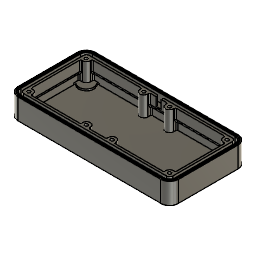
Case Bottom (Autodesk Fusion 360 design; units mm, degrees)
Autodesk Fusion 360 part; units mm, degrees
sketch "Sketch1" plane through (0, 0, 0) normal (0, 0, 1) x (1, 0, 0)
  line L0 (2, 0) -> (146, 0)
  line L1 (148, 2) -> (148, 62)
  line L2 (146, 64) -> (2, 64)
  line L3 (0, 62) -> (0, 2)
  arc A0 (2, 64) -> (0, 62) centre (2, 62) ccw
  arc A1 (0, 2) -> (2, 0) centre (2, 2) ccw
  arc A2 (146, 0) -> (148, 2) centre (146, 2) ccw
  arc A3 (148, 62) -> (146, 64) centre (146, 62) ccw
  line L4 (-0.4, 62) -> (-0.4, 2)
  arc A4 (-0.4, 2) -> (2, -0.4) centre (2, 2) ccw
  line L5 (2, -0.4) -> (146, -0.4)
  arc A5 (146, -0.4) -> (148.4, 2) centre (146, 2) ccw
  line L6 (148.4, 2) -> (148.4, 62)
  arc A6 (148.4, 62) -> (146, 64.4) centre (146, 62) ccw
  line L7 (146, 64.4) -> (2, 64.4)
  arc A7 (2, 64.4) -> (-0.4, 62) centre (2, 62) ccw
  circle A8 centre (3, 61) radius 4
  circle A9 centre (61, 61) radius 4
  circle A10 centre (87, 61) radius 4
  circle A11 centre (3, 3) radius 4
  circle A12 centre (61, 3) radius 4
  circle A13 centre (87, 3) radius 4
  circle A14 centre (145, 3) radius 4
  circle A15 centre (145, 61) radius 4
  line L8 (7, 61) -> (7, 64.4)
  line L9 (3, 57) -> (-0.4, 57)
  line L10 (57, 61) -> (57, 62)
  line L11 (57, 62) -> (57, 64.4)
  line L12 (65, 61) -> (65, 62.4151)
  line L13 (65, 62.4151) -> (65, 64.4)
  line L14 (83, 61) -> (83, 64.4)
  line L15 (91, 61) -> (91, 64.4)
  line L16 (141, 61) -> (141, 64.4)
  line L17 (145, 57) -> (148.4, 57)
  line L18 (145, 7) -> (148.4, 7)
  line L19 (141, 3) -> (141, -0.4)
  line L20 (91, 3) -> (91, -0.4)
  line L21 (83, 3) -> (83, -0.4)
  line L22 (65, 3) -> (65, -0.4)
  line L23 (57, 3) -> (57, -0.4)
  line L24 (7, 3) -> (7, -0.4)
  line L25 (3, 7) -> (-0.4, 7)
  line L26 (-7, 62) -> (-7, 2)
  arc A16 (-7, 2) -> (2, -7) centre (2, 2) ccw
  line L27 (2, -7) -> (146, -7)
  arc A17 (146, -7) -> (155, 2) centre (146, 2) ccw
  line L28 (155, 2) -> (155, 62)
  arc A18 (155, 62) -> (146, 71) centre (146, 62) ccw
  line L29 (146, 71) -> (2, 71)
  arc A19 (2, 71) -> (-7, 62) centre (2, 62) ccw
  point P0 (148, 0)
  point P1 (0, 64)
  point P2 (3, 61)
  point P3 (3, 3)
  point P4 (61, 3)
  point P5 (87, 3)
  point P6 (145, 3)
  point P7 (61, 61)
  point P8 (87, 61)
  point P9 (145, 61)
  dimension "d1" = 148
  dimension "d2" = 64
  dimension "d3" = 2
  dimension "d4" = 0.4
  dimension "d5" = 3
  dimension "d6" = 3
  dimension "d7" = 3
  dimension "d8" = 58
  dimension "d9" = 3
  dimension "d10" = 58
  dimension "d11" = 3
  dimension "d12" = 3
  dimension "d13" = 3
  dimension "d14" = 3
  dimension "d15" = 3
  dimension "d16" = 3
  dimension "d17" = 58
  dimension "d18" = 3
  dimension "d19" = 3
  dimension "d20" = 58
  dimension "d21" = 8
  dimension "d22" = 8
  dimension "d23" = 8
  dimension "d24" = 8
  dimension "d25" = 8
  dimension "d26" = 8
  dimension "d27" = 8
  dimension "d28" = 8
  dimension "d96" = 7
  constraint horizontal L0
  constraint vertical L1
  constraint horizontal L2
  constraint vertical L3
  constraint coincident P1 L3
  constraint coincident P1 L2
  constraint tangent L3 A0
  constraint tangent L2 A0
  constraint coincident origin L3
  constraint coincident origin L0
  constraint tangent L3 A1
  constraint tangent L0 A1
  constraint equal A0 A1
  constraint coincident P0 L1
  constraint coincident P0 L0
  constraint tangent L1 A2
  constraint tangent L0 A2
  constraint equal A0 A2
  constraint tangent L1 A3
  constraint tangent L2 A3
  constraint equal A0 A3
  constraint coincident P2 A8.centre
  constraint coincident P7 A9.centre
  constraint coincident P8 A10.centre
  constraint coincident P3 A11.centre
  constraint coincident P4 A12.centre
  constraint coincident P5 A13.centre
  constraint coincident P6 A14.centre
  constraint coincident P9 A15.centre
  constraint coincident A8 L8.start
  constraint coincident L7 L8.end
  constraint perpendicular L7 L8
  constraint tangent A8 L8
  constraint coincident A8 L9.start
  constraint coincident L4 L9.end
  constraint perpendicular L4 L9
  constraint tangent A8 L9
  constraint coincident A9 L10.start
  constraint tangent A9 L10
  constraint perpendicular L9 L10
  constraint coincident L7 L11.end
  constraint perpendicular L7 L11
  constraint coincident A9 L12.start
  constraint tangent A9 L12
  constraint perpendicular L7 L12
  constraint coincident L7 L13.end
  constraint perpendicular L7 L13
  constraint coincident A10 L14.start
  constraint coincident L7 L14.end
  constraint perpendicular L7 L14
  constraint coincident A10 L15.start
  constraint coincident L7 L15.end
  constraint perpendicular L7 L15
  constraint tangent A10 L14
  constraint tangent A10 L15
  constraint coincident A15 L16.start
  constraint coincident L7 L16.end
  constraint perpendicular L7 L16
  constraint coincident A15 L17.start
  constraint coincident L6 L17.end
  constraint perpendicular L6 L17
  constraint tangent A15 L16
  constraint tangent A15 L17
  constraint coincident A14 L18.start
  constraint coincident L6 L18.end
  constraint tangent A14 L18
  constraint coincident A14 L19.start
  constraint coincident L5 L19.end
  constraint perpendicular L5 L19
  constraint coincident A13 L20.start
  constraint coincident L5 L20.end
  constraint perpendicular L5 L20
  constraint coincident A13 L21.start
  constraint coincident L5 L21.end
  constraint perpendicular L5 L21
  constraint tangent A13 L20
  constraint tangent A13 L21
  constraint tangent A14 L19
  constraint perpendicular L6 L18
  constraint coincident A12 L22.start
  constraint coincident L5 L22.end
  constraint perpendicular L5 L22
  constraint coincident A12 L23.start
  constraint coincident L5 L23.end
  constraint perpendicular L5 L23
  constraint tangent A12 L22
  constraint tangent A12 L23
  constraint coincident A11 L24.start
  constraint coincident L5 L24.end
  constraint perpendicular L5 L24
  constraint coincident A11 L25.start
  constraint coincident L4 L25.end
  constraint perpendicular L4 L25
  constraint tangent A11 L25
  constraint tangent A11 L24
  measures "d1" distance of origin P0
  measures "d2" distance of origin P1
  measures "d3" radius of A0
  measures "d5" distance of L3 P2
  measures "d6" distance of L2 P2
  measures "d7" distance of L2 P7
  measures "d8" distance of P2 P7
  measures "d9" distance of L2 P8
  measures "d10" horizontal distance of P8 P9
  measures "d11" distance of L2 P9
  measures "d12" distance of L1 P9
  measures "d13" distance of L0 P6
  measures "d14" distance of L1 P6
  measures "d15" distance of L0 P5
  measures "d16" distance of L0 P4
  measures "d17" horizontal distance of P3 P4
  measures "d18" distance of L3 P3
  measures "d19" distance of L0 P3
  measures "d20" distance of P5 P6
  measures "d21" diameter of A8
  measures "d22" diameter of A9
  measures "d23" diameter of A10
  measures "d24" diameter of A11
  measures "d25" diameter of A12
  measures "d26" diameter of A13
  measures "d27" diameter of A14
  measures "d28" diameter of A15
extrude "Extrude1" add sketch "Sketch1" along normal blind 20 contours L0 L3 A1 A11 | L0 L3 A1 L4 A4 L5 A11 | L0 A11 L24 | L0 L5 A11 L24 | L4 A4 L5 A11 | L3 L4 A11 L25 | L3 A11 L25 | L0 A12 L23 | L0 L5 A12 L23 | L0 A12 | L0 L5 A12 | L3 L4 A8 L9 | L3 A8 L9 | L0 A12 L22 | L0 L5 A12 L22 | L5 A12 | L2 L3 A0 L4 L7 A7 A8 | L2 L3 A0 A8 | L4 L7 A7 A8 | L2 A8 L8 | L0 A13 L21 | L0 L5 A13 L21 | L2 L7 A8 L8 | L0 A13 | L0 L5 A13 | L2 L7 A9 L11 | L2 A9 L10 L11 | L0 A13 L20 | L0 L5 A13 L20 | L5 A13 | L2 L7 A9 | L2 A9 | L7 A9 | L2 L7 A9 L13 | L2 A9 L12 L13 | L0 A14 L19 | L0 L5 A14 L19 | L0 L1 A2 A14 | L0 L1 A2 L5 A5 L6 A14 | L2 L7 A10 L14 | L2 A10 L14 | L5 A5 L6 A14 | L1 A14 L18 | L2 L7 A10 | L2 A10 | L1 L6 A14 L18 | L7 A10 | L2 L7 A10 L15 | L2 A10 L15 | L1 A15 L17 | L1 L6 A15 L17 | L1 L2 A3 A15 | L1 L2 A3 L6 A6 L7 A15 | L2 L7 A15 L16 | L2 A15 L16 | L6 A6 L7 A15 | L26 A16 L27 A17 L28 A18 L29 A19
sketch "PCB Reference" plane through (0, 0, 20) normal (0, 0, 1) x (-1, 0, 0)
  line L0 (-7, 0.4) -> (-7, -3)
  arc A0 (-7, -3) -> (-3, -7) centre (-3, -3) ccw
  line L1 (-3, -7) -> (0.4, -7)
  line L2 (0.4, -7) -> (0.4, -57)
  line L3 (0.4, -57) -> (-3, -57)
  arc A1 (-3, -57) -> (-7, -61) centre (-3, -61) ccw
  line L4 (-7, -61) -> (-7, -64.4)
  line L5 (-7, -64.4) -> (-57, -64.4)
  line L6 (-57, -64.4) -> (-57, -61)
  arc A2 (-57, -61) -> (-65, -61) centre (-61, -61) ccw
  line L7 (-65, -61) -> (-65, -64.4)
  line L8 (-65, -64.4) -> (-83, -64.4)
  line L9 (-83, -64.4) -> (-83, -61)
  arc A3 (-83, -61) -> (-91, -61) centre (-87, -61) ccw
  line L10 (-91, -61) -> (-91, -64.4)
  line L11 (-91, -64.4) -> (-141, -64.4)
  line L12 (-141, 0.4) -> (-91, 0.4)
  line L13 (-91, 0.4) -> (-91, -3)
  arc A4 (-91, -3) -> (-83, -3) centre (-87, -3) ccw
  line L14 (-83, -3) -> (-83, 0.4)
  line L15 (-83, 0.4) -> (-65, 0.4)
  line L16 (-65, 0.4) -> (-65, -3)
  arc A5 (-65, -3) -> (-57, -3) centre (-61, -3) ccw
  line L17 (-57, -3) -> (-57, 0.4)
  line L18 (-57, 0.4) -> (-7, 0.4)
  line L19 (-2, -64) -> (-146, -64)
  line L20 (-148, -62) -> (-148, -2)
  line L21 (-146, 0) -> (-2, 0)
  line L22 (0, -2) -> (0, -62)
  arc A6 (-2, -64) -> (0, -62) centre (-2, -62) ccw
  arc A7 (0, -2) -> (-2, 0) centre (-2, -2) ccw
  arc A8 (-146, 0) -> (-148, -2) centre (-146, -2) ccw
  arc A9 (-148, -62) -> (-146, -64) centre (-146, -62) ccw
  arc A10 (-148.4, -62) -> (-146, -64.4) centre (-146, -62) ccw
  line L23 (-2, -64.4) -> (-146, -64.4)
  arc A11 (-2, -64.4) -> (0.4, -62) centre (-2, -62) ccw
  line L24 (0.4, -2) -> (0.4, -62)
  arc A12 (0.4, -2) -> (-2, 0.4) centre (-2, -2) ccw
  line L25 (-146, 0.4) -> (-2, 0.4)
  arc A13 (-146, 0.4) -> (-148.4, -2) centre (-146, -2) ccw
  line L26 (-148.4, -62) -> (-148.4, -2)
  line L27 (6.4, -70.4) -> (-154.4, -70.4)
  line L28 (-154.4, -70.4) -> (-154.4, 6.4)
  line L29 (-154.4, 6.4) -> (6.4, 6.4)
  line L30 (6.4, 6.4) -> (6.4, -70.4)
  line L31 (-141, -64.4) -> (-141, -61)
  arc A14 (-141, -61) -> (-145, -57) centre (-145, -61) ccw
  line L32 (-145, -57) -> (-148.4, -57)
  line L33 (-148.4, -57) -> (-148.4, -7)
  line L34 (-148.4, -7) -> (-145, -7)
  arc A15 (-145, -7) -> (-141, -3) centre (-145, -3) ccw
  line L35 (-141, -3) -> (-141, 0.4)
  arc A16 (-2, -71) -> (7, -62) centre (-2, -62) ccw
  line L36 (7, -62) -> (7, -2)
  arc A17 (7, -2) -> (-2, 7) centre (-2, -2) ccw
  line L37 (-2, 7) -> (-146, 7)
  arc A18 (-146, 7) -> (-155, -2) centre (-146, -2) ccw
  line L38 (-155, -2) -> (-155, -62)
  arc A19 (-155, -62) -> (-146, -71) centre (-146, -62) ccw
  line L39 (-146, -71) -> (-2, -71)
  point P0 (0, -64)
  point P1 (-148, -64)
  dimension "d36" = 64.8
  dimension "d37" = 148
  dimension "d38" = 64
  dimension "d39" = 0.4
  dimension "d40" = 0.4
  dimension "d41" = 2
  dimension "d42" = -0.4
  constraint horizontal L19
  constraint vertical L20
  constraint horizontal L21
  constraint vertical L22
  constraint coincident P0 L19
  constraint coincident P0 L22
  constraint tangent L19 A6
  constraint tangent L22 A6
  constraint coincident origin L22
  constraint coincident origin L21
  constraint tangent L22 A7
  constraint tangent L21 A7
  constraint equal A6 A7
  constraint tangent L21 A8
  constraint tangent L20 A8
  constraint equal A6 A8
  constraint coincident P1 L20
  constraint coincident P1 L19
  constraint tangent L20 A9
  constraint tangent L19 A9
  constraint equal A6 A9
  constraint horizontal L27
  constraint vertical L28
  constraint horizontal L29
  constraint vertical L30
  measures "d36" distance of L5 L18
  measures "d37" distance of P0 P1
  measures "d38" distance of P0 origin
  measures "d39" distance of L5 L19
  measures "d40" distance of L2 L22
  measures "d41" radius of A6
sketch "Sketch3" plane through (0, 0, 20) normal (0, 0, 1) x (-1, 0, 0)
  line L0 (-7, -64.4) -> (-57, -64.4)
  line L1 (0.4, -7) -> (0.4, -57)
  line L2 (0.4, -57) -> (-3, -57)
  arc A0 (-3, -57) -> (-7, -61) centre (-3, -61) ccw
  line L3 (-7, -61) -> (-7, -64.4)
  circle A1 centre (-3, -61) radius 2
  circle A2 centre (-61, -61) radius 2
  arc A3 (-57, -61) -> (-65, -61) centre (-61, -61) ccw
  circle A4 centre (-87, -61) radius 2
  arc A5 (-83, -61) -> (-91, -61) centre (-87, -61) ccw
  circle A6 centre (-145, -61) radius 2
  arc A7 (-141, -61) -> (-145, -57) centre (-145, -61) ccw
  circle A8 centre (-145, -3) radius 2
  arc A9 (-145, -7) -> (-141, -3) centre (-145, -3) ccw
  circle A10 centre (-87, -3) radius 2
  arc A11 (-91, -3) -> (-83, -3) centre (-87, -3) ccw
  circle A12 centre (-61, -3) radius 2
  arc A13 (-65, -3) -> (-57, -3) centre (-61, -3) ccw
  circle A14 centre (-3, -3) radius 2
  arc A15 (-7, -3) -> (-3, -7) centre (-3, -3) ccw
  line L4 (-7, 0.4) -> (-7, -3)
  arc A16 (-7, -3) -> (-3, -7) centre (-3, -3) ccw
  line L5 (-3, -7) -> (0.4, -7)
  line L6 (-57, -64.4) -> (-57, -61)
  arc A17 (-57, -61) -> (-65, -61) centre (-61, -61) ccw
  line L7 (-65, -61) -> (-65, -64.4)
  line L8 (-65, -64.4) -> (-83, -64.4)
  line L9 (-83, -64.4) -> (-83, -61)
  arc A18 (-83, -61) -> (-91, -61) centre (-87, -61) ccw
  line L10 (-91, -61) -> (-91, -64.4)
  line L11 (-91, -64.4) -> (-141, -64.4)
  line L12 (-141, -64.4) -> (-141, -61)
  arc A19 (-141, -61) -> (-145, -57) centre (-145, -61) ccw
  line L13 (-145, -57) -> (-148.4, -57)
  line L14 (-148.4, -57) -> (-148.4, -7)
  line L15 (-148.4, -7) -> (-145, -7)
  arc A20 (-145, -7) -> (-141, -3) centre (-145, -3) ccw
  line L16 (-141, -3) -> (-141, 0.4)
  line L17 (-141, 0.4) -> (-91, 0.4)
  line L18 (-91, 0.4) -> (-91, -3)
  arc A21 (-91, -3) -> (-83, -3) centre (-87, -3) ccw
  line L19 (-83, -3) -> (-83, 0.4)
  line L20 (-83, 0.4) -> (-65, 0.4)
  line L21 (-65, 0.4) -> (-65, -3)
  arc A22 (-65, -3) -> (-57, -3) centre (-61, -3) ccw
  line L22 (-57, -3) -> (-57, 0.4)
  line L23 (-57, 0.4) -> (-7, 0.4)
  arc A23 (-2, -71) -> (7, -62) centre (-2, -62) ccw
  line L24 (7, -62) -> (7, -2)
  arc A24 (7, -2) -> (-2, 7) centre (-2, -2) ccw
  line L25 (-2, 7) -> (-146, 7)
  arc A25 (-146, 7) -> (-155, -2) centre (-146, -2) ccw
  line L26 (-155, -2) -> (-155, -62)
  arc A26 (-155, -62) -> (-146, -71) centre (-146, -62) ccw
  line L27 (-146, -71) -> (-2, -71)
  dimension "d49" = 4
  dimension "d50" = 4
  dimension "d51" = 4
  dimension "d52" = 4
  dimension "d53" = 4
  dimension "d54" = 4
  dimension "d55" = 4
  dimension "d56" = 4
  constraint concentric A0 A1
  constraint concentric A2 A3
  constraint concentric A4 A5
  constraint concentric A6 A7
  constraint concentric A8 A9
  constraint concentric A10 A11
  constraint concentric A12 A13
  constraint concentric A14 A15
  measures "d49" diameter of A1
  measures "d50" diameter of A2
  measures "d51" diameter of A4
  measures "d52" diameter of A6
  measures "d53" diameter of A8
  measures "d54" diameter of A10
  measures "d55" diameter of A12
  measures "d56" diameter of A14
hole "Hole1" at (3, 61, 20) at (61, 61, 20) at (87, 61, 20) at (61, 3, 20) at (87, 3, 20) at (3, 3, 20) at (145, 3, 20) at (145, 61, 20) direction (0, 0, -1) diameter 2.5 depth 6 tip angle 180 countersink diameter 3.2 countersink angle 12
sketch "Sketch4" plane through (0, 0, 20) normal (0, 0, 1) x (-1, 0, 0)
  line L0 (-7, -64.4) -> (-57, -64.4)
  line L1 (0.4, -7) -> (0.4, -57)
  line L2 (0.4, -57) -> (-3, -57)
  arc A0 (-3, -57) -> (-7, -61) centre (-3, -61) ccw
  line L3 (-7, -61) -> (-7, -64.4)
  line L4 (-7, -64.4) -> (-57, -64.4)
  line L5 (-57, -64.4) -> (-57, -62.9)
  line L6 (-57, -62.9) -> (-7, -62.9)
  line L7 (-7, -62.9) -> (-7, -64.4)
  line L8 (-65, -64.4) -> (-83, -64.4)
  line L9 (-83, -64.4) -> (-83, -62.9)
  line L10 (-83, -62.9) -> (-65, -62.9)
  line L11 (-65, -62.9) -> (-65, -64.4)
  line L12 (-91, -64.4) -> (-141, -64.4)
  line L13 (-141, -64.4) -> (-141, -62.9)
  line L14 (-141, -62.9) -> (-91, -62.9)
  line L15 (-91, -62.9) -> (-91, -64.4)
  line L16 (-148.4, -57) -> (-146.9, -57)
  line L17 (-146.9, -57) -> (-146.9, -7)
  line L18 (-146.9, -7) -> (-148.4, -7)
  line L19 (-148.4, -7) -> (-148.4, -57)
  arc A1 (-145, -7) -> (-141, -3) centre (-145, -3) ccw
  line L20 (-141, 0.4) -> (-91, 0.4)
  line L21 (-91, 0.4) -> (-91, -1.1)
  line L22 (-91, -1.1) -> (-141, -1.1)
  line L23 (-141, -1.1) -> (-141, 0.4)
  line L24 (-83, 0.4) -> (-65, 0.4)
  line L25 (-65, 0.4) -> (-65, -1.1)
  line L26 (-65, -1.1) -> (-83, -1.1)
  line L27 (-83, -1.1) -> (-83, 0.4)
  line L28 (-57, 0.4) -> (-7, 0.4)
  line L29 (-7, 0.4) -> (-7, -1.1)
  line L30 (-7, -1.1) -> (-57, -1.1)
  line L31 (-57, -1.1) -> (-57, 0.4)
  line L32 (0.4, -7) -> (-1.1, -7)
  line L33 (-1.1, -7) -> (-1.1, -57)
  line L34 (-1.1, -57) -> (0.4, -57)
  line L35 (0.4, -57) -> (0.4, -7)
  circle A2 centre (-145, -3) radius 1.6
  circle A3 centre (-87, -3) radius 1.6
  circle A4 centre (-87, -61) radius 1.6
  circle A5 centre (-3, -61) radius 1.6
  circle A6 centre (-61, -61) radius 1.6
  circle A7 centre (-61, -3) radius 1.6
  circle A8 centre (-3, -3) radius 1.6
  circle A9 centre (-145, -61) radius 1.6
  line L36 (-7, 0.4) -> (-7, -3)
  arc A10 (-7, -3) -> (-3, -7) centre (-3, -3) ccw
  line L37 (-3, -7) -> (0.4, -7)
  line L38 (-57, -64.4) -> (-57, -61)
  arc A11 (-57, -61) -> (-65, -61) centre (-61, -61) ccw
  line L39 (-65, -61) -> (-65, -64.4)
  line L40 (-65, -64.4) -> (-83, -64.4)
  line L41 (-83, -64.4) -> (-83, -61)
  arc A12 (-83, -61) -> (-91, -61) centre (-87, -61) ccw
  line L42 (-91, -61) -> (-91, -64.4)
  line L43 (-91, -64.4) -> (-141, -64.4)
  line L44 (-141, -64.4) -> (-141, -61)
  arc A13 (-141, -61) -> (-145, -57) centre (-145, -61) ccw
  line L45 (-145, -57) -> (-148.4, -57)
  line L46 (-148.4, -57) -> (-148.4, -7)
  line L47 (-148.4, -7) -> (-145, -7)
  arc A14 (-145, -7) -> (-141, -3) centre (-145, -3) ccw
  line L48 (-141, -3) -> (-141, 0.4)
  line L49 (-141, 0.4) -> (-91, 0.4)
  line L50 (-91, 0.4) -> (-91, -3)
  arc A15 (-91, -3) -> (-83, -3) centre (-87, -3) ccw
  line L51 (-83, -3) -> (-83, 0.4)
  line L52 (-83, 0.4) -> (-65, 0.4)
  line L53 (-65, 0.4) -> (-65, -3)
  arc A16 (-65, -3) -> (-57, -3) centre (-61, -3) ccw
  line L54 (-57, -3) -> (-57, 0.4)
  line L55 (-57, 0.4) -> (-7, 0.4)
  arc A17 (-2, -71) -> (7, -62) centre (-2, -62) ccw
  line L56 (7, -62) -> (7, -2)
  arc A18 (7, -2) -> (-2, 7) centre (-2, -2) ccw
  line L57 (-2, 7) -> (-146, 7)
  arc A19 (-146, 7) -> (-155, -2) centre (-146, -2) ccw
  line L58 (-155, -2) -> (-155, -62)
  arc A20 (-155, -62) -> (-146, -71) centre (-146, -62) ccw
  line L59 (-146, -71) -> (-2, -71)
  point P0 (-65, -64.4)
  point P1 (-91, -64.4)
  point P2 (-148.4, -57)
  point P3 (-141, 0.4)
  point P4 (-83, 0.4)
  point P5 (-57, 0.4)
  point P6 (0.4, -7)
  dimension "d62" = 1.5
  dimension "d63" = 1.5
  dimension "d64" = 1.5
  dimension "d65" = 1.5
  dimension "d66" = 1.5
  dimension "d67" = 1.5
  dimension "d68" = 1.5
  dimension "d69" = 1.5
  constraint horizontal L4
  constraint vertical L5
  constraint horizontal L6
  constraint vertical L7
  constraint coincident L0.start L3.end
  constraint horizontal L8
  constraint vertical L9
  constraint horizontal L10
  constraint vertical L11
  constraint coincident P0 L8.start
  constraint horizontal L12
  constraint vertical L13
  constraint horizontal L14
  constraint vertical L15
  constraint coincident P1 L12.start
  constraint horizontal L16
  constraint vertical L17
  constraint horizontal L18
  constraint vertical L19
  constraint coincident P2 L16.start
  constraint horizontal L20
  constraint vertical L21
  constraint horizontal L22
  constraint vertical L23
  constraint coincident P3 L20.start
  constraint horizontal L24
  constraint vertical L25
  constraint horizontal L26
  constraint vertical L27
  constraint coincident P4 L24.start
  constraint horizontal L28
  constraint vertical L29
  constraint horizontal L30
  constraint vertical L31
  constraint coincident P5 L28.start
  constraint horizontal L32
  constraint vertical L33
  constraint horizontal L34
  constraint vertical L35
  constraint coincident P6 L1.start
  measures "d62" distance of L0.start L6.end
  measures "d63" distance of P0 L10.end
  measures "d64" distance of P1 L14.end
  measures "d65" distance of P2 L16.end
  measures "d66" distance of P3 L22.end
  measures "d67" distance of P4 L26.end
  measures "d68" distance of P5 L30.end
  measures "d69" distance of P6 L32.end
extrude "Extrude3" add sketch "Sketch4" 1 faces at (71, -4.8, 20) against normal blind 13 contours L0 L3 L4 L5 L6 L7 L38 | L1 L2 L32 L33 L34 L35 L37 | L8 L9 L10 L11 L39 L40 L41 | L28 L29 L30 L31 L36 L54 L55 | L12 L13 L14 L15 L42 L43 L44 | L24 L25 L26 L27 L51 L52 L53 | L16 L17 L18 L19 L45 L46 L47 | L20 L21 L22 L23 L48 L49 L50
chamfer "Chamfer1" distance 1.5 distance2 3 8 edges at (32, 62.9, 7) (74, 62.9, 7) (116, 62.9, 7) (1.1, 32, 7) (32, 1.1, 7) (74, 1.1, 7) (116, 1.1, 7) (146.9, 32, 7) measured on face at (23.6667, 63.9, 7) measured on face at (77, 63.9, 7) measured on face at (124.3333, 63.9, 7) measured on face at (0.1, 23.6667, 7) measured on face at (40.3333, 0.6, 7) measured on face at (71, 0.1, 7) measured on face at (124.3333, 0.1, 7) measured on face at (147.9, 40.3333, 7)
sketch "Sketch5" plane through (0, 0, 20) normal (0, 0, 1) x (-1, 0, 0)
  line L0 (-7, -62.9) -> (-57, -62.9)
  line L1 (-57, -62.9) -> (-57, -61)
  arc A0 (-57, -61) -> (-65, -61) centre (-61, -61) ccw
  line L2 (-65, -61) -> (-65, -62.9)
  line L3 (-65, -62.9) -> (-83, -62.9)
  circle A1 centre (-61, -61) radius 1.6
  line L4 (-71.5, -65.2) -> (-76.5, -65.2)
  line L5 (-76.5, -65.2) -> (-76.5, -62.4)
  line L6 (-76.5, -62.4) -> (-71.5, -62.4)
  line L7 (-71.5, -62.4) -> (-71.5, -65.2)
  line L8 (-141, -62.9) -> (-141, -61)
  arc A2 (-141, -61) -> (-145, -57) centre (-145, -61) ccw
  line L9 (-145, -57) -> (-146.9, -57)
  line L10 (-146.9, -57) -> (-146.9, -7)
  line L11 (-146.9, -7) -> (-145, -7)
  arc A3 (-145, -7) -> (-141, -3) centre (-145, -3) ccw
  line L12 (-141, -3) -> (-141, -1.1)
  line L13 (-141, -1.1) -> (-91, -1.1)
  line L14 (-91, -1.1) -> (-91, -3)
  arc A4 (-91, -3) -> (-83, -3) centre (-87, -3) ccw
  line L15 (-83, -3) -> (-83, -1.1)
  line L16 (-83, -1.1) -> (-65, -1.1)
  line L17 (-65, -1.1) -> (-65, -3)
  arc A5 (-65, -3) -> (-57, -3) centre (-61, -3) ccw
  line L18 (-57, -3) -> (-57, -1.1)
  line L19 (-57, -1.1) -> (-7, -1.1)
  line L20 (-7, -1.1) -> (-7, -3)
  arc A6 (-7, -3) -> (-3, -7) centre (-3, -3) ccw
  line L21 (-3, -7) -> (-1.1, -7)
  line L22 (-1.1, -7) -> (-1.1, -57)
  line L23 (-1.1, -57) -> (-3, -57)
  arc A7 (-3, -57) -> (-7, -61) centre (-3, -61) ccw
  line L24 (-7, -61) -> (-7, -62.9)
  line L25 (-83, -62.9) -> (-83, -61)
  arc A8 (-83, -61) -> (-91, -61) centre (-87, -61) ccw
  line L26 (-91, -61) -> (-91, -62.9)
  line L27 (-91, -62.9) -> (-141, -62.9)
  circle A9 centre (-145, -3) radius 1.6
  circle A10 centre (-87, -3) radius 1.6
  circle A11 centre (-87, -61) radius 1.6
  circle A12 centre (-3, -61) radius 1.6
  circle A13 centre (-61, -3) radius 1.6
  circle A14 centre (-3, -3) radius 1.6
  circle A15 centre (-145, -61) radius 1.6
  arc A16 (-2, -71) -> (7, -62) centre (-2, -62) ccw
  line L28 (7, -62) -> (7, -2)
  arc A17 (7, -2) -> (-2, 7) centre (-2, -2) ccw
  line L29 (-2, 7) -> (-146, 7)
  arc A18 (-146, 7) -> (-155, -2) centre (-146, -2) ccw
  line L30 (-155, -2) -> (-155, -62)
  arc A19 (-155, -62) -> (-146, -71) centre (-146, -62) ccw
  line L31 (-146, -71) -> (-2, -71)
  line L32 (1.2, -62) -> (1.2, -2)
  arc A20 (1.2, -2) -> (-2, 1.2) centre (-2, -2) ccw
  line L33 (-2, 1.2) -> (-146, 1.2)
  arc A21 (-146, 1.2) -> (-149.2, -2) centre (-146, -2) ccw
  line L34 (-149.2, -2) -> (-149.2, -62)
  arc A22 (-149.2, -62) -> (-146, -65.2) centre (-146, -62) ccw
  line L35 (-146, -65.2) -> (-2, -65.2)
  arc A23 (-2, -65.2) -> (1.2, -62) centre (-2, -62) ccw
  line L36 (4, -62) -> (4, -2)
  arc A24 (4, -2) -> (-2, 4) centre (-2, -2) ccw
  line L37 (-2, 4) -> (-146, 4)
  arc A25 (-146, 4) -> (-152, -2) centre (-146, -2) ccw
  line L38 (-152, -2) -> (-152, -62)
  arc A26 (-152, -62) -> (-146, -68) centre (-146, -62) ccw
  line L39 (-146, -68) -> (-2, -68)
  arc A27 (-2, -68) -> (4, -62) centre (-2, -62) ccw
  dimension "d84" = 5
  dimension "d85" = 6.5
  dimension "d97" = -5.8
  dimension "d98" = -3
  constraint horizontal L4
  constraint vertical L5
  constraint horizontal L6
  constraint vertical L7
  measures "d84" distance of L4.start L4.end
  measures "d85" horizontal distance of L2.end L4.start
extrude "Extrude4" cut sketch "Sketch5" against normal blind 8.5 contours L3 L4 L5 L7 L35 | L3 L5 L6 L7 | L36 A24 L37 A25 L38 A26 L39 A27
chamfer "Chamfer2" distance 1 angle 45 2 edges at (71.5, 65.2, 15.75) (76.5, 65.2, 15.75)
sketch "Sketch8" plane through (0, 0, 20) normal (0, 0, 1) x (-1, 0, 0)
  line L0 (4, -2) -> (4, -62)
  arc A0 (-2, -68) -> (4, -62) centre (-2, -62) ccw
  line L1 (-2, -68) -> (-146, -68)
  arc A1 (-152, -62) -> (-146, -68) centre (-146, -62) ccw
  line L2 (-152, -62) -> (-152, -2)
  arc A2 (-146, 4) -> (-152, -2) centre (-146, -2) ccw
  line L3 (-146, 4) -> (-2, 4)
  arc A3 (4, -2) -> (-2, 4) centre (-2, -2) ccw
  arc A4 (-2, -71) -> (7, -62) centre (-2, -62) ccw
  line L4 (7, -62) -> (7, -2)
  arc A5 (7, -2) -> (-2, 7) centre (-2, -2) ccw
  line L5 (-2, 7) -> (-146, 7)
  arc A6 (-146, 7) -> (-155, -2) centre (-146, -2) ccw
  line L6 (-155, -2) -> (-155, -62)
  arc A7 (-155, -62) -> (-146, -71) centre (-146, -62) ccw
  line L7 (-146, -71) -> (-2, -71)
  line L8 (5.8, -62) -> (5.8, -2)
  arc A8 (5.8, -2) -> (-2, 5.8) centre (-2, -2) ccw
  line L9 (-2, 5.8) -> (-146, 5.8)
  arc A9 (-146, 5.8) -> (-153.8, -2) centre (-146, -2) ccw
  line L10 (-153.8, -2) -> (-153.8, -62)
  arc A10 (-153.8, -62) -> (-146, -69.8) centre (-146, -62) ccw
  line L11 (-146, -69.8) -> (-2, -69.8)
  arc A11 (-2, -69.8) -> (5.8, -62) centre (-2, -62) ccw
  line L12 (5, -62) -> (5, -2)
  arc A12 (5, -2) -> (-2, 5) centre (-2, -2) ccw
  line L13 (-2, 5) -> (-146, 5)
  arc A13 (-146, 5) -> (-153, -2) centre (-146, -2) ccw
  line L14 (-153, -2) -> (-153, -62)
  arc A14 (-153, -62) -> (-146, -69) centre (-146, -62) ccw
  line L15 (-146, -69) -> (-2, -69)
  arc A15 (-2, -69) -> (5, -62) centre (-2, -62) ccw
  dimension "d99" = -1.2
  dimension "d100" = -2
extrude "Extrude6" add sketch "Sketch8" along normal blind 0.6 contours L8 A8 L9 A9 L10 A10 L11 A11
sketch "Sketch9" plane through (0, 0, 0) normal (0, 0, -1) x (1, 0, 0)
  line L0 (7, -3) -> (7, 0.4)
  line L1 (7, 0.4) -> (57, 0.4)
  line L2 (57, 0.4) -> (57, -3)
  arc A0 (57, -3) -> (65, -3) centre (61, -3) ccw
  line L3 (65, -3) -> (65, 0.4)
  line L4 (65, 0.4) -> (83, 0.4)
  line L5 (83, 0.4) -> (83, -3)
  arc A1 (83, -3) -> (91, -3) centre (87, -3) ccw
  line L6 (91, -3) -> (91, 0.4)
  line L7 (91, 0.4) -> (141, 0.4)
  line L8 (141, 0.4) -> (141, -3)
  arc A2 (141, -3) -> (145, -7) centre (145, -3) ccw
  line L9 (145, -7) -> (148.4, -7)
  line L10 (148.4, -7) -> (148.4, -57)
  line L11 (148.4, -57) -> (145, -57)
  arc A3 (145, -57) -> (141, -61) centre (145, -61) ccw
  line L12 (141, -61) -> (141, -64.4)
  line L13 (141, -64.4) -> (91, -64.4)
  line L14 (91, -64.4) -> (91, -61)
  arc A4 (91, -61) -> (83, -61) centre (87, -61) ccw
  line L15 (83, -61) -> (83, -64.4)
  line L16 (83, -64.4) -> (65, -64.4)
  line L17 (65, -64.4) -> (65, -61)
  arc A5 (65, -61) -> (57, -61) centre (61, -61) ccw
  line L18 (57, -61) -> (57, -64.4)
  line L19 (57, -64.4) -> (7, -64.4)
  line L20 (7, -64.4) -> (7, -61)
  arc A6 (7, -61) -> (3, -57) centre (3, -61) ccw
  line L21 (3, -57) -> (-0.4, -57)
  line L22 (-0.4, -57) -> (-0.4, -7)
  line L23 (-0.4, -7) -> (3, -7)
  arc A7 (3, -7) -> (7, -3) centre (3, -3) ccw
  arc A8 (-7, -62) -> (2, -71) centre (2, -62) ccw
  line L24 (2, -71) -> (146, -71)
  arc A9 (146, -71) -> (155, -62) centre (146, -62) ccw
  line L25 (155, -62) -> (155, -2)
  arc A10 (155, -2) -> (146, 7) centre (146, -2) ccw
  line L26 (146, 7) -> (2, 7)
  arc A11 (2, 7) -> (-7, -2) centre (2, -2) ccw
  line L27 (-7, -2) -> (-7, -62)
  line L28 (2, 7) -> (146, 7)
  line L29 (155, -2) -> (155, -62)
  line L30 (146, -71) -> (2, -71)
  line L31 (-7, -62) -> (-7, -2)
  arc A12 (2, 7) -> (-7, -2) centre (2, -2) ccw
  arc A13 (-7, -62) -> (2, -71) centre (2, -62) ccw
  arc A14 (146, -71) -> (155, -62) centre (146, -62) ccw
  arc A15 (155, -2) -> (146, 7) centre (146, -2) ccw
  dimension "d103" = 9
  constraint horizontal L28
  constraint vertical L29
  constraint horizontal L30
  constraint vertical L31
  constraint tangent L28 A12
  constraint tangent L31 A12
  constraint tangent L30 A13
  constraint tangent L31 A13
  constraint equal A12 A13
  constraint tangent L29 A14
  constraint tangent L30 A14
  constraint equal A12 A14
  constraint tangent L28 A15
  constraint tangent L29 A15
  constraint equal A12 A15
  measures "d103" radius of A12
extrude "Extrude7" add sketch "Sketch9" along normal blind 2 contours L0 L1 L2 A0 L3 L4 L5 A1 L6 L7 L8 A2 L9 L10 L11 A3 L12 L13 L14 A4 L15 L16 L17 A5 L18 L19 L20 A6 L21 L22 L23 A7 | A8 L24 A9 L25 A10 L26 A11 L27 L28 L29 L30 L31 A12 A13 A14 A15
fillet "Fillet4" radius 1 8 edges at (-4.364, 68.364, -2) (74, 71, -2) (152.364, 68.364, -2) (155, 32, -2) (152.364, -4.364, -2) (74, -7, -2) (-4.364, -4.364, -2) (-7, 32, -2)
sketch "Sketch10" plane through (0, 0, -2) normal (0, 0, -1) x (1, 0, 0)
  arc A0 (-6, -62) -> (2, -70) centre (2, -62) ccw
  line L0 (2, -70) -> (146, -70)
  arc A1 (146, -70) -> (154, -62) centre (146, -62) ccw
  line L1 (154, -62) -> (154, -2)
  arc A2 (154, -2) -> (146, 6) centre (146, -2) ccw
  line L2 (146, 6) -> (2, 6)
  arc A3 (2, 6) -> (-6, -2) centre (2, -2) ccw
  line L3 (-6, -2) -> (-6, -62)
  circle A4 centre (6, -6) radius 6
  circle A5 centre (6, -58) radius 6
  line L4 (2, 7) -> (146, 7)
  line L5 (74, 7) -> (74, -70)
  circle A6 centre (142, -6) radius 6
  circle A7 centre (142, -58) radius 6
  point P0 (2, -2)
  point P1 (2, -62)
  point P2 (2, -62)
  dimension "d108" = 12
  dimension "d109" = 12
  dimension "d110" = 4
  dimension "d111" = 4
  dimension "d112" = 4
  dimension "d113" = 4
  constraint midpoint L4 L5.start
  constraint midpoint L0 L5.end
  constraint symmetric A4 L5 A6
  constraint symmetric A5 L5 A7
  measures "d108" diameter of A4
  measures "d109" diameter of A5
  measures "d110" horizontal distance of A4.centre P0
  measures "d111" vertical distance of A4.centre P0
  measures "d112" horizontal distance of A5.centre P2
  measures "d113" vertical distance of A5.centre P2
extrude "Extrude8" cut sketch "Sketch10" against normal blind 3 contours A4 | A5 | A6 | A7
sketch "Sketch11" plane through (0, 0, 0) normal (0, 0, 1) x (-1, 0, 0)
  arc A0 (-0.0839, -57) -> (-7, -63.9161) centre (-6, -58) ccw
  line L0 (-0.0839, -57) -> (0.4, -57)
  line L1 (0.4, -57) -> (0.4, -7)
  line L2 (0.4, -7) -> (-0.0839, -7)
  arc A1 (-7, -0.0839) -> (-0.0839, -7) centre (-6, -6) ccw
  line L3 (-7, -0.0839) -> (-7, 0.4)
  line L4 (-7, 0.4) -> (-57, 0.4)
  line L5 (-57, 0.4) -> (-57, -3)
  arc A2 (-65, -3) -> (-57, -3) centre (-61, -3) ccw
  line L6 (-65, -3) -> (-65, 0.4)
  line L7 (-65, 0.4) -> (-83, 0.4)
  line L8 (-83, 0.4) -> (-83, -3)
  arc A3 (-91, -3) -> (-83, -3) centre (-87, -3) ccw
  line L9 (-91, -3) -> (-91, 0.4)
  line L10 (-91, 0.4) -> (-141, 0.4)
  line L11 (-141, 0.4) -> (-141, -0.0839)
  arc A4 (-147.9161, -7) -> (-141, -0.0839) centre (-142, -6) ccw
  line L12 (-147.9161, -7) -> (-148.4, -7)
  line L13 (-148.4, -7) -> (-148.4, -57)
  line L14 (-148.4, -57) -> (-147.9161, -57)
  arc A5 (-141, -63.9161) -> (-147.9161, -57) centre (-142, -58) ccw
  line L15 (-141, -63.9161) -> (-141, -64.4)
  line L16 (-141, -64.4) -> (-91, -64.4)
  line L17 (-91, -64.4) -> (-91, -61)
  arc A6 (-83, -61) -> (-91, -61) centre (-87, -61) ccw
  line L18 (-83, -61) -> (-83, -64.4)
  line L19 (-83, -64.4) -> (-65, -64.4)
  line L20 (-65, -64.4) -> (-65, -61)
  arc A7 (-57, -61) -> (-65, -61) centre (-61, -61) ccw
  line L21 (-57, -61) -> (-57, -64.4)
  line L22 (-57, -64.4) -> (-7, -64.4)
  line L23 (-7, -64.4) -> (-7, -63.9161)
  circle A8 centre (-6, -58) radius 7.5
  circle A9 centre (-6, -6) radius 7.5
  circle A10 centre (-142, -58) radius 7.5
  circle A11 centre (-142, -6) radius 7.5
  dimension "d116" = 15
  dimension "d117" = 15
  dimension "d118" = 15
  dimension "d119" = 15
  constraint concentric A0 A8
  constraint concentric A1 A9
  constraint concentric A5 A10
  constraint concentric A4 A11
  measures "d116" diameter of A8
  measures "d117" diameter of A9
  measures "d118" diameter of A10
  measures "d119" diameter of A11
extrude "Extrude9" add sketch "Sketch11" along normal blind 1.6 contours A0 L0 L1 L22 L23 A8 | A0 L0 L1 L22 L23 A8 | L1 L2 A1 L3 L4 A9 | L1 L2 A1 L3 L4 A9 | L13 L14 A5 L15 L16 A10 | L13 L14 A5 L15 L16 A10 | L10 L11 A4 L12 L13 A11 | L10 L11 A4 L12 L13 A11
fillet "Fillet5" radius 1 8 edges at (9.9102, 64.4, 0.8) (138.0898, 64.4, 0.8) (148.4, 54.0898, 0.8) (148.4, 9.9102, 0.8) (138.0898, -0.4, 0.8) (9.9102, -0.4, 0.8) (-0.4, 9.9102, 0.8) (-0.4, 54.0898, 0.8)
fillet "Fillet6" radius 1 48 edges at (57, 63.65, 8.5) (57, 62.9, 15) (57, 64.4, 3.5) (83, 62.9, 15) (83, 63.65, 8.5) (83, 64.4, 3.5) (146.9, 57, 15) (148.4, 57, 4.3) (147.65, 57, 8.5) (141, 64.4, 4.3) (141, 63.65, 8.5) (141, 62.9, 15) (7, 62.9, 15) (1.1, 57, 15) (0.35, 57, 8.5) (-0.4, 57, 4.3) (7, 64.4, 4.3) (7, 63.65, 8.5) (65, 64.4, 3.5) (65, 63.65, 8.5) (65, 62.9, 15) (91, 62.9, 15) (91, 63.65, 8.5) (91, 64.4, 3.5) (1.1, 7, 15) (7, 1.1, 15) (7, 0.35, 8.5) (7, -0.4, 4.3) (-0.4, 7, 4.3) (0.35, 7, 8.5) (65, 1.1, 15) (65, 0.35, 8.5) (65, -0.4, 3.5) (91, 1.1, 15) (91, 0.35, 8.5) (91, -0.4, 3.5) (146.9, 7, 15) (147.65, 7, 8.5) (148.4, 7, 4.3) (141, -0.4, 4.3) (141, 0.35, 8.5) (141, 1.1, 15) (83, 1.1, 15) (83, 0.35, 8.5) (83, -0.4, 3.5) (57, 1.1, 15) (57, 0.35, 8.5) (57, -0.4, 3.5)
equation "d85 = ( ( 18 - 5 ) / 2 ) * 1 mm"
equation "d120 = ( 0.4 * 4 ) * 1 mm"
